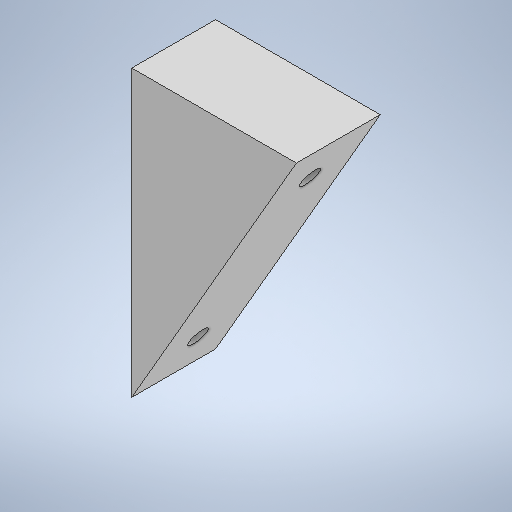
# Autodesk Inventor part: face 30°
Saved by Autodesk Inventor 2026.2 (Build 302298010, 298A)
## iProperties
Created: 2026-05-12
Part Number: face 30°
Material: Générique
Document SubType Name: Modeling
Designer: Genon
Density: 1 g/cm^3
Appearance: Par défaut
Author: Genon
Autodesk Inventor part; units mm, degrees
ref_plane "YZ Plane" through (0, 0, 0) normal (1, 0, 0) x (0, 1, 0)
ref_plane "XZ Plane" through (0, 0, 0) normal (0, 1, 0) x (-1, 0, 0)
ref_plane "XY Plane" through (0, 0, 0) normal (0, 0, 1) x (1, 0, 0)
sketch "Esquisse1" plane through (0, 0, 0) normal (1, 0, 0) x (0, 1, 0)
  line L0 (0, 0) -> (25, 0)
  line L1 (25, 0) -> (25, -7.347)
  line L2 (25, -7.347) -> (0, -7.347)
  line L3 (0, -7.347) -> (0, 0)
  dimension "d0" = 25
  dimension "d1" = 7.347
  constraints: 8 end point, 2 parallel, 1 horizontal, 1 perpendicular
  measures "d0" distance of L1.end L2.end
  measures "d1" distance of L0.end L1.end
extrude "Extrusion1" add sketch "Esquisse1" along normal blind 20
sketch "Esquisse3" plane through (20, 0, 0) normal (1, 0, 0) x (0, 0, -1)
  line L0 (0, 0) -> (7.347, 0) projected
  line L1 (0, 0) -> (3.5, 0)
  line L2 (3.5, 0) -> (3.5, 4)
  line L3 (7.347, 25) -> (0, 25) projected
  line L4 (0, 25) -> (3.5, 25)
  line L5 (3.5, 25) -> (3.5, 21)
  dimension "d7" = 3.5
  dimension "d8" = 4
  dimension "d9" = 3.5
  dimension "d10" = 4
  dimension "d11" = 90
  constraints: 8 end point, 2 coincident, 2 perpendicular, 2 point on line
  measures "d7" distance of L0.start L1.end
  measures "d8" distance of L1.end L2.end
  measures "d9" distance of L3.end L4.end
  measures "d10" distance of L4.end L5.end
  measures "d11" angle of L4 L5
hole "Perçage1" at (20, 4, -3.5) at (20, 21, -3.5) direction (-1, 0, 0) diameter 1.6 end through all
sketch "Esquisse4" plane through (0, 0, 0) normal (0, 0, 1) x (1, 0, 0)
  line L0 (0, 0) -> (20, 0) projected
  line L1 (0, 0) -> (14.4338, 25)
  line L2 (0, 25) -> (20, 25) projected
  line L3 (0, 0) -> (28.8675, 0) construction
  line L4 (0, 25) -> (20, 25) projected
  line L5 (20, 25) -> (20, 0) projected
  point P0 (10, 17.3205)
  dimension "d19" = 60
  constraints: 4 end point, 1 equal length, 1 horizontal, 1 point on line
  measures "d19" angle of L3 L1
extrude "Extrusion3" cut sketch "Esquisse4" against normal blind 10
